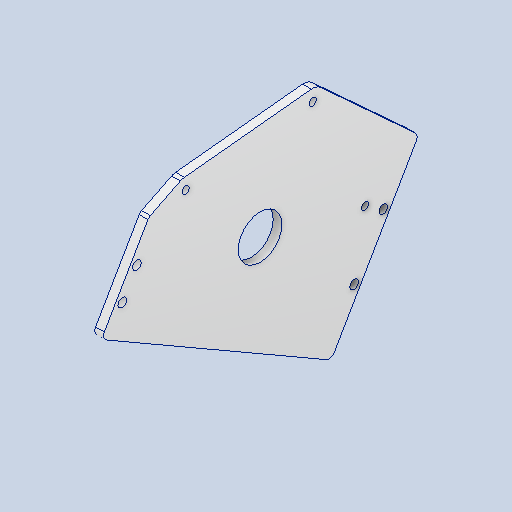
# Autodesk Inventor part: belt_liner_v5_Plate_1
Saved by Autodesk Inventor 2025.2 (Build 292293000, 293)
## iProperties
Created: 2025-02-22
Part Number: belt_liner_v5_Plate_1
Material: アルミニウム 6061
Document SubType Name: Modeling
Designer: haruy
Density: 2.7 g/cm^3
Appearance: アルミニウム - フラット
Author: haruy
Autodesk Inventor part; units mm, degrees
ref_plane "YZ Plane" through (0, 0, 0) normal (1, 0, 0) x (0, 1, 0)
ref_plane "XZ Plane" through (0, 0, 0) normal (0, 1, 0) x (-1, 0, 0)
ref_plane "XY Plane" through (0, 0, 0) normal (0, 0, 1) x (1, 0, 0)
derived "belt_liner_v5_Sketch_Base.ipt"
sketch "スケッチ1" plane through (300, 0, 0) normal (1, 0, 0) x (0, 1, 0)
  circle A0 centre (0, 0) radius 22.36 construction
  circle A1 centre (742.4003, -428.625) radius 23.875 construction
  line L0 (0, 0) -> (0, -985.832) projected
  line L1 (0, 0) -> (742.4003, -428.625) projected
  line L2 (-48.7433, -24.4258) -> (-56.2433, -37.4162) projected
  line L3 (-56.2433, -37.4162) -> (725.7777, -488.9162) projected
  line L4 (725.7777, -488.9162) -> (733.2777, -475.9258) projected
  line L5 (733.2777, -475.9258) -> (-48.7433, -24.4258) projected
  line L6 (-44.1225, 123.2584) -> (-44.1225, 123.2584) projected
  line L7 (0, -985.832) -> (0, 0) projected
  circle A2 centre (0, 0) radius 12.5 construction
  circle A3 centre (0, 0) radius 15 construction
  line L8 (0, 0) -> (0, 0) projected
  circle A4 centre (0, 0) radius 24.06 construction
  line L9 (0, 0) -> (0, 0) projected
  line L10 (0, 0) -> (0, 0) projected
  line L11 (-48.7433, -24.4258) -> (-46.2433, -20.0957) projected
  circle A5 centre (742.4003, -428.625) radius 5 projected
  line L12 (733.2777, -475.9258) -> (707.2969, -460.9258) projected
  line L13 (707.2969, -460.9258) -> (709.7969, -456.5957) projected
  line L14 (709.7969, -456.5957) -> (735.7777, -471.5957) projected
  line L15 (735.7777, -471.5957) -> (733.2777, -475.9258) projected
  circle A6 centre (738.0702, -426.125) radius 5.1 projected
  line L16 (742.4003, -428.625) -> (509.0943, -293.9257) projected
  circle A7 centre (759.7208, -438.625) radius 5.1 projected
  line L17 (740.6202, -421.7083) -> (762.2708, -434.2083) projected
  line L18 (735.5202, -430.5417) -> (757.1708, -443.0417) projected
  circle A8 centre (742.4003, -428.625) radius 22.175 construction
  circle A9 centre (738.0702, -426.125) radius 10.1 construction
  circle A10 centre (759.7208, -438.625) radius 10.1 construction
  line L19 (743.1202, -417.3781) -> (764.7708, -429.8781) construction
  line L20 (733.0202, -434.8719) -> (754.6708, -447.3719) construction
  line L21 (743.1202, -417.3781) -> (730.6598, -410.1842) construction
  line L22 (729.3233, -421.075) -> (734.3733, -412.3281) construction
  line L23 (764.7708, -429.8781) -> (770.9335, -433.4362) construction
  line L24 (770.9335, -433.4362) -> (771.2695, -433.6302) projected
  line L25 (754.6708, -447.3719) -> (764.7708, -429.8781) projected
  line L26 (764.7708, -429.8781) -> (773.431, -434.8781) projected
  line L27 (773.431, -434.8781) -> (763.331, -452.3719) projected
  line L28 (763.331, -452.3719) -> (754.6708, -447.3719) construction
  circle A11 centre (725.8674, -468.7607) radius 1.5 projected
  circle A12 centre (0, 0) radius 30 construction
  circle A13 centre (742.4003, -428.625) radius 6 construction
  circle A14 centre (0, 0) radius 24.06 construction
  circle A15 centre (0, 0) radius 24.06 construction
  circle A16 centre (742.4003, -428.625) radius 24.06 projected
  line L29 (754.4303, -407.7884) -> (12.03, 20.8366) construction
  circle A17 centre (725.8592, -419.075) radius 4 projected
  circle A18 centre (725.8592, -419.075) radius 1.5 projected
  circle A19 centre (742.4003, -428.625) radius 18.525 construction
  circle A20 centre (748.9869, -417.4167) radius 4 projected
  line L30 (737.4369, -437.4219) -> (742.4869, -428.675) projected
  circle A21 centre (748.9869, -417.4167) radius 1.5 projected
  line L31 (734.3733, -412.3281) -> (737.8233, -406.3526) construction
  line L32 (737.8233, -406.3526) -> (776.881, -428.9026) projected
  line L33 (773.431, -434.8781) -> (776.881, -428.9026) projected
  line L34 (737.8233, -406.3526) -> (723.6503, -415.7402) projected
  line L35 (720.8233, -435.7974) -> (759.881, -458.3474) projected
  line L36 (720.8233, -435.7974) -> (721.8667, -418.8295) projected
  line L37 (763.331, -452.3719) -> (759.881, -458.3474) projected
  circle A22 centre (735.9869, -439.9333) radius 4 projected
  circle A23 centre (735.9869, -439.9333) radius 1.5 projected
  circle A24 centre (717.2072, -463.7607) radius 1.5 projected
  circle A25 centre (742.4003, -428.625) radius 34.06 projected
  circle A26 centre (742.4869, -428.675) radius 8.5 projected
  line L38 (-57.9836, -13.421) -> (-72.9836, -13.421) projected
  line L39 (-72.9836, -13.421) -> (-72.9836, -353.421) projected
  line L40 (-72.9836, -353.421) -> (-57.9836, -353.421) projected
  line L41 (-57.9836, -353.421) -> (-57.9836, -13.421) projected
  line L42 (457.0164, -338.421) -> (-72.9836, -338.421) projected
  line L43 (-72.9836, -338.421) -> (-72.9836, -353.421) projected
  line L44 (-72.9836, -353.421) -> (457.0164, -353.421) projected
  line L45 (457.0164, -353.421) -> (457.0164, -338.421) projected
  line L46 (427.0164, -338.421) -> (427.0164, -353.421) projected
  line L47 (457.0164, -353.421) -> (491.0931, -353.421) projected
  line L48 (491.0931, -353.421) -> (498.5931, -340.4306) projected
  line L49 (246.7786, -212.3659) -> (254.2786, -199.3755) projected
  line L50 (-207.9836, 176.579) -> (-227.9836, 176.579) projected
  line L51 (-227.9836, 176.579) -> (-227.9836, -413.421) projected
  line L52 (-227.9836, -413.421) -> (-207.9836, -413.421) projected
  line L53 (-207.9836, -413.421) -> (-207.9836, 176.579) projected
  line L54 (-52.0815, -339.4226) -> (-53.6411, -349.3003) projected
  line L55 (-53.6411, -349.3003) -> (703.9845, -468.9194) projected
  line L56 (703.9845, -468.9194) -> (705.5441, -459.0417) projected
  line L57 (705.5441, -459.0417) -> (-52.0815, -339.4226) projected
  circle A27 centre (0, 0) radius 24.06 construction
  line L58 (1412.7204, 281.579) -> (-606.6364, 281.579) projected
  line L59 (1185.5776, -518.421) -> (-909.402, -518.421) projected
  line L60 (9.7721, 46.9258) -> (885.3238, -458.5742) projected
  line L61 (885.3238, -458.5742) -> (892.8238, -445.5838) projected
  line L62 (892.8238, -445.5838) -> (17.2721, 59.9162) projected
  line L63 (17.2721, 59.9162) -> (9.7721, 46.9258) projected
  line L64 (32.4276, 51.1662) -> (872.4722, -433.8338) projected
  line L65 (872.4722, -433.8338) -> (876.2222, -427.3386) projected
  line L66 (876.2222, -427.3386) -> (36.1776, 57.6614) projected
  line L67 (36.1776, 57.6614) -> (32.4276, 51.1662) projected
  line L68 (36.1776, 57.6614) -> (94.8941, 23.7614) projected
  line L69 (94.8941, 23.7614) -> (97.6441, 28.5245) projected
  line L70 (97.6441, 28.5245) -> (38.9276, 62.4245) projected
  line L71 (38.9276, 62.4245) -> (36.1776, 57.6614) projected
  circle A28 centre (215.5519, 104.2106) radius 120 projected
  line L72 (-37.9836, 123.579) -> (-57.9836, 123.579) projected
  line L73 (-57.9836, 123.579) -> (-57.9836, 103.579) projected
  line L74 (-57.9836, 103.579) -> (-37.9836, 103.579) projected
  line L75 (-37.9836, 103.579) -> (-37.9836, 123.579) projected
  line L76 (215.5519, 104.2106) -> (184.4936, 220.1217) projected
  line L77 (215.5519, 104.2106) -> (99.6408, 73.1523) projected
  line L78 (215.5519, 104.2106) -> (155.5519, 0.2876) projected
  line L79 (187.4936, 225.3179) -> (96.6408, 67.9562) projected
  line L80 (96.6408, 67.9562) -> (91.4447, 70.9562) projected
  line L81 (91.4447, 70.9562) -> (182.2975, 228.3179) projected
  line L82 (182.2975, 228.3179) -> (187.4936, 225.3179) projected
  line L83 (182.2975, 228.3179) -> (179.2975, 223.1217) projected
  line L84 (179.2975, 223.1217) -> (174.9674, 225.6217) projected
  line L85 (174.9674, 225.6217) -> (177.9674, 230.8179) projected
  line L86 (177.9674, 230.8179) -> (182.2975, 228.3179) projected
  line L87 (91.4447, 70.9562) -> (94.4447, 76.1523) projected
  line L88 (94.4447, 76.1523) -> (90.1146, 78.6523) projected
  line L89 (90.1146, 78.6523) -> (87.1146, 73.4562) projected
  line L90 (87.1146, 73.4562) -> (91.4447, 70.9562) projected
  line L91 (-37.9836, 123.579) -> (2.0164, 123.579) projected
  line L92 (2.0164, 123.579) -> (2.0164, 103.579) projected
  line L93 (2.0164, 103.579) -> (-37.9836, 103.579) projected
  line L94 (-37.9836, 103.579) -> (-37.9836, 123.579) projected
  circle A29 centre (215.5519, 104.2106) radius 132.0681 projected
  line L95 (101.1776, 170.2447) -> (38.9276, 62.4245) projected
  line L96 (32.4276, 51.1662) -> (11.6951, 15.2564) construction
  line L97 (11.6951, 15.2564) -> (20.3553, 10.2564) construction
  line L98 (20.3553, 10.2564) -> (41.0878, 46.1662) construction
  line L99 (41.0878, 46.1662) -> (32.4276, 51.1662) projected
  line L100 (149.5179, -10.1638) -> (155.5519, 0.2876) projected
  line L101 (149.5179, -10.1638) -> (20.3553, 10.2564) construction
  line L102 (79.4739, 0.91) -> (82.9739, 6.9722) projected
  line L103 (82.9739, 6.9722) -> (98.7532, -2.138) projected
  line L104 (179.2975, 223.1217) -> (151.7911, 205.8696) projected
  line L105 (94.4447, 76.1523) -> (95.6322, 108.5996) projected
  line L106 (96.6408, 67.9562) -> (113.8929, 40.4498) projected
  line L107 (-324.9836, 281.579) -> (-324.9836, -518.421) projected
  line L108 (1175.0164, 281.579) -> (1175.0164, -518.421) projected
  line L109 (17.2721, 59.9162) -> (9.7721, 46.9258) projected
  line L110 (9.7721, 46.9258) -> (-3.2183, 54.4258) projected
  line L111 (-3.2183, 54.4258) -> (4.2817, 67.4162) projected
  line L112 (4.2817, 67.4162) -> (17.2721, 59.9162) projected
  line L113 (-3.2183, 54.4258) -> (-5.7183, 50.0957) projected
  line L114 (-5.7183, 50.0957) -> (22.4276, 33.8457) projected
  line L115 (22.4276, 33.8457) -> (24.9276, 38.1758) projected
  line L116 (24.9276, 38.1758) -> (-3.2183, 54.4258) projected
  line L117 (-48.7433, -24.4258) -> (-46.2433, -20.0957) projected
  line L118 (-46.2433, -20.0957) -> (5.7183, -50.0957) projected
  line L119 (5.7183, -50.0957) -> (3.2183, -54.4258) projected
  line L120 (3.2183, -54.4258) -> (-48.7433, -24.4258) projected
  line L121 (789.6086, -403.313) -> (798.2689, -408.313) projected
  line L122 (798.2689, -408.313) -> (785.0364, -431.2324) projected
  line L123 (785.0364, -431.2324) -> (776.3761, -426.2324) projected
  line L124 (776.3761, -426.2324) -> (789.6086, -403.313) projected
  line L125 (885.3238, -458.5742) -> (882.8238, -462.9043) projected
  line L126 (882.8238, -462.9043) -> (856.843, -447.9043) projected
  line L127 (856.843, -447.9043) -> (859.343, -443.5742) projected
  line L128 (859.343, -443.5742) -> (885.3238, -458.5742) projected
  line L129 (7.6071, 48.1758) -> (11.9372, 45.6758) projected
  line L130 (11.9372, 45.6758) -> (19.4372, 58.6662) projected
  line L131 (19.4372, 58.6662) -> (15.1071, 61.1662) projected
  line L132 (15.1071, 61.1662) -> (7.6071, 48.1758) projected
  line L133 (19.4372, 58.6662) -> (14.4372, 50.0059) projected
  line L134 (14.4372, 50.0059) -> (24.8295, 44.0059) projected
  line L135 (24.8295, 44.0059) -> (29.8295, 52.6662) projected
  line L136 (29.8295, 52.6662) -> (19.4372, 58.6662) projected
  line L137 (931.2231, -485.0742) -> (935.5533, -487.5742) projected
  line L138 (935.5533, -487.5742) -> (951.5533, -459.8614) projected
  line L139 (951.5533, -459.8614) -> (947.2231, -457.3614) projected
  line L140 (947.2231, -457.3614) -> (931.2231, -485.0742) projected
  line L141 (944.4731, -462.1245) -> (934.9731, -478.579) projected
  line L142 (934.9731, -478.579) -> (919.3847, -469.579) projected
  line L143 (919.3847, -469.579) -> (928.8847, -453.1245) projected
  line L144 (928.8847, -453.1245) -> (944.4731, -462.1245) projected
  line L145 (924.1347, -461.3518) -> (939.7231, -470.3518) projected
  line L146 (926.6347, -457.0216) -> (921.6347, -465.6819) projected
  line L147 (921.6347, -465.6819) -> (882.6635, -443.1819) projected
  line L148 (882.6635, -443.1819) -> (887.6635, -434.5216) projected
  line L149 (887.6635, -434.5216) -> (926.6347, -457.0216) projected
  line L150 (888.9135, -432.3566) -> (881.4135, -445.347) projected
  line L151 (881.4135, -445.347) -> (874.4853, -441.347) projected
  line L152 (874.4853, -441.347) -> (881.9853, -428.3566) projected
  line L153 (881.9853, -428.3566) -> (888.9135, -432.3566) projected
  line L154 (31.0795, 54.8313) -> (23.5795, 41.8409) projected
  line L155 (23.5795, 41.8409) -> (30.5077, 37.8409) projected
  line L156 (30.5077, 37.8409) -> (38.0077, 50.8313) projected
  line L157 (38.0077, 50.8313) -> (31.0795, 54.8313) projected
  line L158 (16.9372, 54.3361) -> (27.3295, 48.3361) projected
  circle A30 centre (4.192, 47.2607) radius 1.25 projected
  circle A31 centre (12.8522, 42.2607) radius 1.25 projected
  line L159 (17.2721, 59.9162) -> (9.7721, 46.9258) projected
  line L160 (885.3238, -458.5742) -> (882.8238, -462.9043) projected
  line L161 (882.8238, -462.9043) -> (933.0533, -491.9043) projected
  line L162 (933.0533, -491.9043) -> (935.5533, -487.5742) projected
  line L163 (935.5533, -487.5742) -> (885.3238, -458.5742) projected
  line L164 (375.0164, 281.579) -> (375.0164, -518.421) projected
  line L165 (38.9276, 62.4245) -> (41.4276, 66.7546) projected
  line L166 (41.4276, 66.7546) -> (100.1441, 32.8546) projected
  line L167 (100.1441, 32.8546) -> (97.6441, 28.5245) projected
  line L168 (97.6441, 28.5245) -> (38.9276, 62.4245) projected
  line L169 (97.7242, 18.6633) -> (115.0447, 8.6633) projected
  line L170 (115.0447, 8.6633) -> (117.5447, 12.9934) projected
  line L171 (117.5447, 12.9934) -> (100.2242, 22.9934) projected
  line L172 (100.2242, 22.9934) -> (97.7242, 18.6633) projected
  line L173 (116.2947, 10.8284) -> (98.9742, 20.8284) projected
  line L174 (457.0164, -338.421) -> (465.1124, -338.421) projected
  line L175 (465.1124, -338.421) -> (472.6124, -325.4306) projected
  line L176 (-48.7433, -24.4258) -> (-56.2433, -37.4162) projected
  line L177 (-56.2433, -37.4162) -> (-77.8939, -24.9162) projected
  line L178 (-77.8939, -24.9162) -> (-70.3939, -11.9258) projected
  line L179 (-70.3939, -11.9258) -> (-48.7433, -24.4258) projected
  line L180 (-207.9836, -73.421) -> (-72.9836, -73.421) projected
  line L181 (-72.9836, -73.421) -> (-72.9836, -93.421) projected
  line L182 (-72.9836, -93.421) -> (-207.9836, -93.421) projected
  line L183 (-207.9836, -93.421) -> (-207.9836, -73.421) projected
  line L184 (-72.9836, -273.421) -> (-207.9836, -273.421) projected
  line L185 (-207.9836, -273.421) -> (-207.9836, -293.421) projected
  line L186 (-207.9836, -293.421) -> (-72.9836, -293.421) projected
  line L187 (-72.9836, -293.421) -> (-72.9836, -273.421) projected
  line L188 (-227.9836, -118.421) -> (-207.9836, -118.421) projected
  circle A32 centre (-30.1728, -32.2607) radius 1.25 construction
  circle A33 centre (-12.8522, -42.2607) radius 1.25 construction
  line L189 (-5.7183, 50.0957) -> (-46.2433, -20.0957) projected
  circle A34 centre (44.6769, 5.3827) radius 15 projected
  circle A35 centre (17.6769, -41.3827) radius 15 projected
  circle A36 centre (44.6769, 5.3827) radius 22 construction
  circle A37 centre (17.6769, -41.3827) radius 22 construction
  circle A38 centre (31.1769, -18) radius 3 projected
  line L190 (44.6769, 5.3827) -> (17.6769, -41.3827) construction
  circle A39 centre (26.7448, 25.5678) radius 3 projected
  circle A40 centre (-8.77, -35.9456) radius 3 projected
  circle A41 centre (0, 0) radius 7.5
  circle A42 centre (26.7448, 25.5678) radius 1.25
  circle A43 centre (31.1769, -18) radius 1.25
  circle A44 centre (-8.77, -35.9456) radius 1.25
  circle A45 centre (26.7448, 25.5678) radius 4
  circle A46 centre (31.1769, -18) radius 4
  line L191 (24.9276, 38.1758) -> (30.3245, 27.3528)
  line L192 (30.7243, 25.9727) -> (35.1564, -17.5952)
  line L193 (34.1258, -20.7026) -> (3.2183, -54.4258)
  circle A47 centre (12.8522, 42.2607) radius 1.5
  circle A48 centre (4.192, 47.2607) radius 1.5
  circle A49 centre (-12.8522, -42.2607) radius 1.5
  circle A50 centre (-30.1728, -32.2607) radius 1.5
  circle A51 centre (866.7533, -450.7393) radius 1.25 projected
  circle A52 centre (875.4135, -455.7393) radius 1.25 projected
  circle A53 centre (992.3767, -344.2894) radius 120 projected
  line L194 (275.5519, 208.1337) -> (1052.3767, -240.3663) projected
  line L195 (-207.9836, -118.421) -> (1175.0164, -118.421) projected
  point P0 (730.6598, -410.1842)
  point P1 (-65.4836, -23.421)
  point P2 (-65.4836, -345.921)
  point P3 (447.0164, -345.921)
  point P4 (437.0164, -345.921)
  point P5 (477.5143, -336.921)
  point P6 (486.1745, -341.921)
  point P7 (-42.9836, -345.921)
  point P8 (694.8867, -462.421)
  point P9 (-57.9836, 113.579)
  point P10 (782.9924, -414.7727)
  point P11 (931.9289, -465.8518)
  point P12 (3.2183, -54.4258)
  point P13 (24.9276, 38.1758)
  dimension "d1" = 15
  dimension "d2" = 2.5
  dimension "d3" = 2.5
  dimension "d4" = 2.5
  dimension "d5" = 8
  dimension "d6" = 8
  dimension "d7" = 3
  dimension "d8" = 3
  dimension "d9" = 3
  dimension "d10" = 3
  constraints: 10 centre point, 10 coincident, 6 end point, 4 point on circle, 4 tangent, 6 other
  measures "d1" diameter of A41
  measures "d2" diameter of A42
  measures "d3" diameter of A43
  measures "d4" diameter of A44
  measures "d5" diameter of A45
  measures "d6" diameter of A46
  measures "d7" diameter of A47
  measures "d8" diameter of A48
  measures "d9" diameter of A49
  measures "d10" diameter of A50
extrude "押し出し1" add sketch "スケッチ1" against normal blind 3 contours A41 L1 A46 L193 A35 L118 L0 | L0 L118 L189 L114 L115 L191 A45 L192 A34 A46 L1 A41 | L118 A35 L119 L5 L0 | L0 L5 L11 L118 | A46 L1 A38 | L1 A38 A46 | A35 L193 L119 L118 | L118 L119 A35 | A38 L1 A43 | L1 A43 A38 | L119 A35 L193 | L113 L110 L60 L115 L114 | A34 L192 | A45 | A39 | A40 picked at (31.8888, 5.1879)
fillet "フィレット1" radius 2 4 edges at (298.5, 24.9276, 38.1758) (298.5, -3.2183, 54.4258) (298.5, -48.7433, -24.4258) (298.5, 3.2183, -54.4258)
